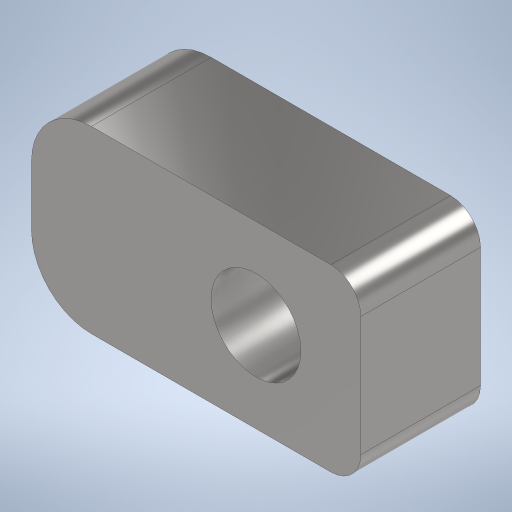
# Autodesk Inventor part: Mocowanie przesuwnicy
Saved by Autodesk Inventor 2024 (Build 280153000, 153)
## iProperties
Created: 2024-04-13
Part Number: Mocowanie przesuwnicy
Material: Stainless Steel
Document SubType Name: Sheet Metal
Designer: HP
Density: 8 g/cm^3
Sheet Metal Rule: Default
Appearance: Semi-Polished
Author: HP
Autodesk Inventor part; units mm, degrees
ref_plane "YZ Plane" through (0, 0, 0) normal (1, 0, 0) x (0, 1, 0)
ref_plane "XZ Plane" through (0, 0, 0) normal (0, 1, 0) x (-1, 0, 0)
ref_plane "XY Plane" through (0, 0, 0) normal (0, 0, 1) x (1, 0, 0)
sketch "Sketch1" plane through (0, 0, 0) normal (0, 0, 1) x (1, 0, 0)
  circle A0 centre (0, 0) radius 3
  line L0 (0, 0) -> (0, 6) construction
  line L1 (0, 6) -> (0, -6) construction
  line L2 (0, -6) -> (5, -6)
  line L3 (7, -4) -> (7, 4)
  line L4 (5, 6) -> (0, 6)
  line L5 (0, 6) -> (-11, 6)
  line L6 (-15, 2) -> (-15, -2)
  line L7 (-11, -6) -> (0, -6)
  arc A1 (7, 4) -> (5, 6) centre (5, 4) ccw
  arc A2 (5, -6) -> (7, -4) centre (5, -4) ccw
  arc A3 (-11, 6) -> (-15, 2) centre (-11, 2) ccw
  arc A4 (-15, -2) -> (-11, -6) centre (-11, -2) ccw
  line L8 (0, 0) -> (9, 0) construction
  line L9 (9, 0) -> (9, 8.7977) construction
  point P0 (7, -6)
  point P1 (-15, 6)
  dimension "d0" = 6
  dimension "d1" = 6
  dimension "d2" = 12
  dimension "d3" = 7
  dimension "d4" = 15
  dimension "d5" = 2
  dimension "d6" = 4
  dimension "d7" = 4
  dimension "d16" = 9
  constraints: 20 end point, 8 point on circle, 8 tangent, 5 centre point, 5 perpendicular, 5 point on line, 2 horizontal, 2 vertical, 1 coincident, 1 equal radius
  measures "d0" diameter of A0
  measures "d1" distance of L0.start L0.end
  measures "d2" distance of L0.end L1.end
  measures "d3" distance of L1.end point (7, -6)
  measures "d4" distance of L0.end point (-15, 6)
  measures "d5" radius of A1
  measures "d6" radius of A3
  measures "d7" radius of A4
  measures "d16" distance of L0.start L8.end
extrude "Extrusion1" add sketch "Sketch1" along normal blind 8
sketch "Sketch3" plane through (-15, -2, 0) normal (-1, 0, 0) x (0, 0, 1)
  line L0 (0, 2) -> (4, 2) construction
  circle A0 centre (4, 2) radius 2.5
  dimension "d17" = 4
  dimension "d18" = 5
  constraints: 2 end point, 1 centre point, 1 coincident, 1 horizontal
  measures "d17" distance of L0.start L0.end
  measures "d18" diameter of A0
extrude "Extrusion3" cut sketch "Sketch3" against normal blind 8
thread "Thread2" size "M5x0.8" class "6H" standard "ANSI Metric M Profile" length 8
equation "\"BendRadius\" = Thickness"
equation "\"BendReliefWidth\" = Thickness"
equation "\"BendReliefDepth\" = 0.5 * Thickness"
equation "\"CornerReliefSize\" = 4 * Thickness"
equation "\"MinimumRemnant\" = 2 * Thickness"
equation "\"TransitionRadius\" = BendRadius"
equation "\"JacobiRadiusSize\" = BendRadius"
equation "\"GapSize\" = Thickness"
equation "\"Thickness\" = 3.048"
body "Solid1"
